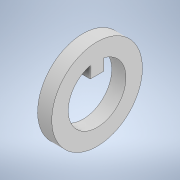
# Autodesk Inventor part: handle insert cover
Saved by Autodesk Inventor 2020.4 (Build 244396000, 396)
## iProperties
Created: 2023-07-18
Part Number: handle insert cover
Material: Generic
Document SubType Name: Modeling
Designer: Paul
Density: 1 g/cm^3
Appearance: Default
Author: Paul
Autodesk Inventor part; units mm, degrees
ref_plane "YZ Plane" through (0, 0, 0) normal (1, 0, 0) x (0, 1, 0)
ref_plane "XZ Plane" through (0, 0, 0) normal (0, 1, 0) x (-1, 0, 0)
ref_plane "XY Plane" through (0, 0, 0) normal (0, 0, 1) x (1, 0, 0)
sketch "Sketch1" plane through (0, 0, 0) normal (1, 0, 0) x (0, 1, 0)
  circle A0 centre (0, 0) radius 6.477
  line L0 (9.271, 1.524) -> (9.271, -1.524)
  line L1 (9.271, -1.524) -> (3.683, -1.524)
  line L2 (3.683, -1.524) -> (3.683, 1.524)
  line L3 (3.683, 1.524) -> (9.271, 1.524)
  line L4 (9.271, 1.524) -> (3.683, -1.524) construction
  line L5 (9.271, -1.524) -> (3.683, 1.524) construction
  circle A1 centre (0, 0) radius 10.16
  line L6 (9.271, 1.524) -> (10.045, 1.524)
  line L7 (9.271, -1.524) -> (10.045, -1.524)
  point P0 (6.477, 0)
  point P1 (6.2952, -1.524)
  point P2 (6.2952, 1.524)
  dimension "d0" = 12.954
  dimension "d1" = 3.048
  dimension "d2" = 5.588
  dimension "d3" = 20.32
  constraints: 16 end point, 3 parallel, 2 coincident, 2 midpoint, 2 perpendicular, 2 point on circle, 1 centre point, 1 vertical, 3 other
  measures "d1" distance of L0.start L0.end
  measures "d2" distance of L0.end L1.end
  measures "d3" diameter of A1
extrude "Extrusion1" add sketch "Sketch1" along normal blind 3.175 contours A0 L1 L2 L3 | A0 L3 L0 L1 | A0 L1 L7 A1 L6 L3 | L6 A1 L7 L0 picked at (4.6143, 0)
body "Solid1"
